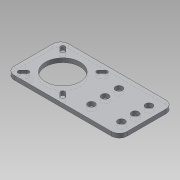
# Autodesk Inventor part: V-Slot Motor Mount Plate
Saved by Autodesk Inventor 2015 (Build 190159000, 159)
## iProperties
Created: 2013-06-20
Part Number: V-Slot Motor Mount Plate
Material: Aluminum 6061
Document SubType Name: Modeling
Designer: Jon Hollander
Density: 2.71 g/cm^3
Mass: 20.5132 g
Surface Area: 64.7141 cm^2
Volume: 7.56944 cm^3
Appearance: Aluminum - Flat
Author: Jon Hollander
Autodesk Inventor part; units mm, degrees
ref_plane "YZ Plane" through (0, 0, 0) normal (1, 0, 0) x (0, 1, 0)
ref_plane "XZ Plane" through (0, 0, 0) normal (0, 1, 0) x (-1, 0, 0)
ref_plane "XY Plane" through (0, 0, 0) normal (0, 0, 1) x (1, 0, 0)
sketch "Sketch1" plane through (0, 0, 0) normal (0, 0, 1) x (1, 0, 0)
  line L0 (-41, -19.75) -> (41, -19.75)
  line L1 (41, -19.75) -> (41, 19.75)
  line L2 (41, 19.75) -> (-41, 19.75)
  line L3 (-41, 19.75) -> (-41, -19.75)
  line L4 (-41, -19.75) -> (41, 19.75) construction
  line L5 (41, -19.75) -> (-41, 19.75) construction
  point P0 (0, 0)
  dimension "d0" = 82
  dimension "d1" = 39.5
  constraints: 12 end point, 2 midpoint, 2 parallel, 1 horizontal, 1 perpendicular
  measures "d0" distance of L2.end L1.end
  measures "d1" distance of L1.end L0.end
extrude "Extrusion1" add sketch "Sketch1" along normal blind 3
sketch "Sketch2" plane through (0, 0, 3) normal (0, 0, 1) x (1, 0, 0)
  line L0 (-41, -19.75) -> (41, -19.75) projected
  line L1 (41, -19.75) -> (41, 19.75) projected
  line L2 (41, 19.75) -> (-41, 19.75) projected
  line L3 (-41, 19.75) -> (-41, -19.75) projected
  line L4 (-41, 0) -> (41, 0) construction
  line L5 (-19.75, 19.75) -> (-19.75, -19.75) construction
  point P0 (0, 0)
  point P1 (-19.75, 0)
  dimension "d4" = 21.25
  constraints: 4 end point, 3 midpoint, 2 point on line, 1 perpendicular
  measures "d4" distance between parallel lines of L3 L5
hole "Hole1" at (-19.75, 0, 3) direction (0, 0, -1) diameter 25 end through all
sketch "Sketch3" plane through (0, 0, 3) normal (0, 0, 1) x (1, 0, 0)
  circle A0 centre (-19.75, 0) radius 12.5 projected
  line L0 (-41, -19.75) -> (41, -19.75) projected
  line L1 (41, 19.75) -> (-41, 19.75) projected
  line L2 (-41, 19.75) -> (-41, -19.75) projected
  line L3 (-19.75, 0) -> (8.1807, 0) construction
  line L4 (-19.75, 0) -> (0, 19.75) construction
  line L5 (-19.75, 0) -> (8.1807, 0) construction
  line L6 (-19.75, 0) -> (0, -19.75) construction
  line L7 (-19.75, 0) -> (-39.5, 19.75) construction
  line L8 (-19.75, 0) -> (-39.5, -19.75) construction
  arc A1 (-31.654, -14.096) -> (-33.846, -11.904) centre (-32.75, -13) ccw
  arc A2 (-36.346, -14.404) -> (-34.154, -16.596) centre (-35.25, -15.5) ccw
  line L9 (-33.846, -11.904) -> (-36.346, -14.404)
  line L10 (-34.154, -16.596) -> (-31.654, -14.096)
  point P0 (0, 0)
  dimension "d13" = 45
  dimension "d14" = 5.75
  dimension "d15" = 8.25
  dimension "d16" = 35.25
  dimension "d17" = 32.75
  dimension "d18" = 3.1
  dimension "d19" = 3.1
  constraints: 16 end point, 4 point on circle, 4 point on line, 4 tangent, 2 centre point, 2 coincident, 2 horizontal, 2 midpoint, 2 perpendicular, 1 collinear, 1 equal length
  measures "d13" angle of L5 L4
  measures "d14" distance from line of L2 point (-35.25, -15.5)
  measures "d15" distance from line of L2 point (-32.75, -13)
  measures "d16" distance from line of L1 point (-35.25, -15.5)
  measures "d17" distance from line of L1 point (-32.75, -13)
  measures "d18" diameter of A1
  measures "d19" diameter of A2
extrude "Extrusion2" cut sketch "Sketch3" against normal through all contours L10 A2 L9 A1
ref_plane "Work Plane1" through (-41, 0, 0) normal (0, 1, 0) x (1, 0, 0)
ref_plane "Work Plane2" through (-19.75, 0, 3) normal (-1, 0, 0) x (0, 0, 1)
mirror "Mirror1" about plane through (-19.75, 0, 3) normal (-1, 0, 0) of "Extrusion2"
mirror "Mirror2" about plane through (-41, 0, 0) normal (0, 1, 0) of "Extrusion2", "Mirror1"
sketch "Sketch4" plane through (0, 0, 3) normal (0, 0, 1) x (1, 0, 0)
  circle A0 centre (-19.75, 0) radius 12.5 projected
  line L0 (-41, -19.75) -> (41, -19.75) projected
  line L1 (41, -19.75) -> (41, 19.75) projected
  line L2 (41, 19.75) -> (-41, 19.75) projected
  line L3 (-41, 19.75) -> (-41, -19.75) projected
  line L4 (11, 19.75) -> (11, -19.75) construction
  line L5 (21.9, 19.75) -> (21.9, -19.75) construction
  line L6 (41, 0) -> (-41, 0) construction
  point P0 (0, 0)
  point P1 (11, 0)
  point P2 (11, 10)
  point P3 (11, -10)
  point P4 (32.8, 0)
  point P5 (32.8, 10)
  point P6 (32.8, -10)
  dimension "d22" = 52
  dimension "d23" = 10.9
  dimension "d24" = 10
  dimension "d25" = 8.2
  dimension "d26" = 9.75
  dimension "d27" = 21.8
  dimension "d28" = 30.75
  constraints: 6 end point, 5 point on line, 4 symmetric about line, 3 midpoint, 2 perpendicular
  measures "d22" distance between parallel lines of L3 L4
  measures "d23" distance between parallel lines of L4 L5
  measures "d24" distance of point (11, 0) point (11, 10)
  measures "d25" distance from line of L1 point (32.8, 0)
  measures "d26" distance from line of L2 point (32.8, 10)
  measures "d27" distance of point (11, 0) point (32.8, 0)
  measures "d28" distance of point (11, 0) A0.centre
hole "Hole2" at (11, 0, 3) at (11, 10, 3) at (11, -10, 3) at (32.8, -10, 3) at (32.8, 10, 3) at (32.8, 0, 3) direction (0, 0, -1) diameter 5.1 end through all
fillet "Fillet1" radius 5.75 4 edges at (-41, 19.75, 1.5) (-41, -19.75, 1.5) (41, -19.75, 1.5) (41, 19.75, 1.5)
equation "\"d19\" = d18"
body "Solid1"
